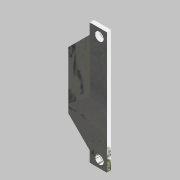
# Autodesk Inventor part: Tritt oben
Saved by Autodesk Inventor 2015 (Build 190159000, 159)
## iProperties
Created: 2017-04-11
Part Number: Tritt oben
Material: Generic
Document SubType Name: Modeling
Designer: Seelenernter
Density: 1 g/cm^3
Appearance: Chrom - poliert
Author: Seelenernter
Autodesk Inventor part; units mm, degrees
ref_plane "YZ Plane" through (0, 0, 0) normal (1, 0, 0) x (0, 1, 0)
sketch "Skizze1" plane through (0, 0, 0) normal (0, 1, 0) x (-1, 0, 0)
  line L0 (-90, 285) -> (90, 285)
  line L1 (90, 285) -> (90, -285)
  line L2 (90, -285) -> (-90, -285)
  line L3 (-90, -285) -> (-90, 285)
  line L4 (-90, 285) -> (90, -285) construction
  line L5 (90, 285) -> (-90, -285) construction
  point P0 (0, 0)
  dimension "d0" = 180
  dimension "d1" = 570
  constraints: 12 end point, 2 midpoint, 2 parallel, 1 horizontal, 1 perpendicular
  measures "d0" distance of L1.end L2.end
  measures "d1" distance of L0.end L1.end
extrude "Extrusion1" add sketch "Skizze1" along normal blind 20
sketch "Skizze2" plane through (0, 20, 0) normal (0, 1, 0) x (1, 0, 0)
  line L0 (-90, -285) -> (90, -285) projected
  line L1 (90, -285) -> (90, 285) projected
  line L2 (90, 285) -> (-90, 285) projected
  line L3 (-90, 285) -> (-90, -285) projected
  circle A0 centre (55, -250) radius 20
  point P0 (0, 0)
  dimension "d4" = 35
  dimension "d5" = 35
  dimension "d6" = 40
  constraints: 1 centre point
  measures "d4" distance from line of L1 A0.centre
  measures "d5" distance from line of L0 A0.centre
  measures "d6" diameter of A0
extrude "Extrusion2" cut sketch "Skizze2" against normal blind 20 contours A0
mirror "Spiegeln1" about plane through (0, 0, 0) normal (0, 0, 1) of "Extrusion2"
sketch "Skizze3" plane through (0, 20, 0) normal (0, 1, 0) x (1, 0, 0)
  circle A0 centre (25, -195) radius 5
  line L0 (-90, -285) -> (90, -285) projected
  line L1 (-90, 285) -> (-90, -285) projected
  circle A1 centre (75, -195) radius 5
  line L2 (90, -285) -> (90, 285) projected
  circle A2 centre (50, -165) radius 5
  circle A3 centre (50, -110) radius 5
  circle A4 centre (50, -55) radius 5
  circle A5 centre (50, 0) radius 5
  circle A6 centre (50, 55) radius 5
  circle A7 centre (50, 110) radius 5
  circle A8 centre (50, 165) radius 5
  circle A9 centre (25, -140) radius 5
  circle A10 centre (75, -140) radius 5
  circle A11 centre (25, -85) radius 5
  circle A12 centre (75, -85) radius 5
  circle A13 centre (25, -30) radius 5
  circle A14 centre (75, -30) radius 5
  circle A15 centre (25, 25) radius 5
  circle A16 centre (75, 25) radius 5
  circle A17 centre (25, 80) radius 5
  circle A18 centre (75, 80) radius 5
  circle A19 centre (25, 135) radius 5
  circle A20 centre (75, 135) radius 5
  circle A21 centre (25, 190) radius 5
  circle A22 centre (75, 190) radius 5
  point P0 (0, 0)
  dimension "d9" = 10
  dimension "d10" = 90
  dimension "d11" = 115
  dimension "d12" = 10
  dimension "d13" = 90
  dimension "d14" = 15
  dimension "d15" = 10
  dimension "d16" = 120
  dimension "d19" = 55
  dimension "d26" = 55
  dimension "d42" = 25
  constraints: 23 centre point, 2 vertical, 40 other
  measures "d9" diameter of A0
  measures "d10" distance from line of L0 A0.centre
  measures "d11" distance from line of A0.centre L1
  measures "d12" diameter of A1
  measures "d13" distance from line of L0 A1.centre
  measures "d14" distance from line of L2 A1.centre
  measures "d15" diameter of A2
  measures "d16" distance from line of L0 A2.centre
  measures "d19" distance of A2.centre A3.centre
  measures "d26" distance of A0.centre A9.centre
  measures "d42" horizontal distance of A1.centre A2.centre
extrude "Extrusion3" add sketch "Skizze3" along normal blind 2
fillet "Rundung1" radius 2 46 edges at (20, 22, 195) (20, 22, 140) (45, 22, 165) (70, 22, 195) (70, 22, 140) (45, 22, 110) (20, 22, 85) (70, 22, 85) (45, 22, 55) (20, 22, 30) (70, 22, 30) (45, 22, 0) (20, 22, -25) (70, 22, -25) (45, 22, -55) (20, 22, -80) (70, 22, -80) (45, 22, -110) (20, 22, -135) (70, 22, -135) (45, 22, -165) (20, 22, -190) (70, 22, -190) (70, 20, -190) (45, 20, -165) (20, 20, -190) (20, 20, -135) (45, 20, -110) (70, 20, -135) (20, 20, -80) (45, 20, -55) (70, 20, -80) (70, 20, -25) (45, 20, 0) (20, 20, -25) (20, 20, 30) (70, 20, 30) (45, 20, 55) (20, 20, 85) (45, 20, 110) (70, 20, 85) (70, 20, 140) (45, 20, 165) (20, 20, 140) (20, 20, 195) (70, 20, 195)
sketch "Skizze4" plane through (0, 20, 0) normal (0, 1, 0) x (1, 0, 0)
  line L0 (90, -285) -> (-90, -285) projected
  line L1 (13, -285) -> (13, 285)
  line L2 (-90, 285) -> (90, 285) projected
  line L3 (15, 285) -> (15, -285)
  point P0 (0, 0)
  dimension "d34" = 103
  dimension "d35" = 2
  constraints: 4 end point, 4 point on line, 1 parallel, 1 vertical
  measures "d34" distance from line of L0.end L1
  measures "d35" distance between parallel lines of L1 L3
extrude "Extrusion4" cut sketch "Skizze4" against normal blind 1
sketch "Skizze5" plane through (-90, 0, 285) normal (0, 0, 1) x (1, 0, 0)
  line L0 (103, 19) -> (103, 20) projected
  line L1 (0, 20) -> (103, 20) projected
  line L2 (0, 0) -> (0, 20) projected
  line L3 (180, 0) -> (0, 0) projected
  line L4 (180, 0) -> (180, 20) projected
  line L5 (105, 20) -> (180, 20) projected
  line L6 (105, 20) -> (105, 19) projected
  line L7 (105, 19) -> (103, 19) projected
  line L8 (103, 19) -> (103, 0)
  line L9 (0, 0) -> (180, 0) projected
  line L10 (105, 19) -> (105, 0)
  point P0 (90, 0)
  constraints: 4 end point, 2 point on line, 1 parallel, 1 vertical
extrude "Extrusion5" cut sketch "Skizze5" against normal blind 1 contours L7 L10 L3 L8
sketch "Skizze6" plane through (90, 0, -285) normal (0, 0, -1) x (-1, 0, 0)
  line L0 (77, 20) -> (77, 19) projected
  line L1 (77, 19) -> (75, 19) projected
  line L2 (75, 19) -> (75, 20) projected
  line L3 (0, 20) -> (75, 20) projected
  line L4 (0, 0) -> (0, 20) projected
  line L5 (180, 0) -> (0, 0) projected
  line L6 (180, 0) -> (180, 20) projected
  line L7 (77, 20) -> (180, 20) projected
  line L8 (75, 19) -> (75, 0)
  line L9 (77, 19) -> (77, 0)
  line L10 (180, 0) -> (0, 0) projected
  point P0 (90, 0)
  constraints: 4 end point, 1 perpendicular, 1 point on line, 1 vertical
extrude "Extrusion6" cut sketch "Skizze6" against normal blind 1 contours L9 L5 L8 L1
sketch "Skizze7" plane through (0, 20, 0) normal (0, 1, 0) x (1, 0, 0)
  line L0 (13, -285) -> (13, 285) projected
  line L1 (13, 285) -> (-90, 285) projected
  line L2 (-90, 285) -> (-90, -285) projected
  line L3 (-90, -285) -> (13, -285) projected
  line L4 (13, -285) -> (-90, -285) projected
  line L5 (10, -285) -> (10, -235)
  line L6 (10, -235) -> (-90, -135)
  line L7 (-90, 285) -> (-90, -285) projected
  line L8 (90, -285) -> (90, 285) projected
  point P0 (0, 0)
  dimension "d43" = 80
  dimension "d44" = 50
  dimension "d45" = 45
  constraints: 4 end point, 2 point on line, 1 parallel
  measures "d43" distance between parallel lines of L8 L5
  measures "d44" distance of L5.start L5.end
  measures "d45" angle of L5 L6
extrude "Extrusion7" cut sketch "Skizze7" against normal blind 20 contours L3 L2 L6 L5
ref_plane "Arbeitsebene1" through (0, 0, 0) normal (0, 0, 1) x (1, 0, 0)
mirror "Spiegeln2" about plane through (0, 0, 0) normal (0, 0, 1) of "Extrusion7"
ref_plane "Arbeitsebene2" through (0, 0, 285) normal (1, 0, 0) x (0, 0, -1)
sketch "Skizze9" plane through (0, 20, 0) normal (0, 1, 0) x (1, 0, 0)
  circle A0 centre (-75, -85) radius 5
  circle A1 centre (-50, -55) radius 5
  circle A2 centre (-25, -85) radius 5
  line L0 (-90, -135) -> (-90, 135) projected
  circle A3 centre (25, -85) radius 3 projected
  circle A4 centre (25, -85) radius 6.4641 projected
  circle A5 centre (50, -55) radius 6.4641 projected
  point P0 (0, 0)
  dimension "d50" = 10
  dimension "d51" = 10
  dimension "d52" = 10
  dimension "d53" = 15
  dimension "d55" = 25
  dimension "d56" = 25
  constraints: 3 centre point, 3 horizontal alignment
  measures "d50" diameter of A0
  measures "d51" diameter of A1
  measures "d52" diameter of A2
  measures "d53" distance from line of L0 A0.centre
  measures "d55" horizontal distance of A0.centre A1.centre
  measures "d56" horizontal distance of A1.centre A2.centre
extrude "Extrusion8" add sketch "Skizze9" along normal blind 2 contours A0 | A1 | A2
fillet "Rundung2" radius 2 6 edges at (-80, 22, 85) (-80, 20, 85) (-55, 22, 55) (-55, 20, 55) (-30, 22, 85) (-30, 20, 85)
pattern_linear "Rechteckige Anordnung1" count 2 spacing 55 along (0, 0, -1) of "Extrusion8", "Rundung2"
mirror "Spiegeln3" about plane through (0, 0, 0) normal (0, 0, 1) of "Extrusion8", "Rundung2"
sketch "Skizze10" plane through (0, 20, 0) normal (0, 1, 0) x (1, 0, 0)
  circle A0 centre (-75, 25) radius 5
  circle A1 centre (-25, 25) radius 5
  circle A2 centre (-50, 55) radius 6.4641 projected
  circle A3 centre (25, 25) radius 6.4641 projected
  circle A4 centre (-25, 85) radius 6.4641 projected
  circle A5 centre (-75, 85) radius 6.4641 projected
  point P0 (0, 0)
  dimension "d63" = 10
  dimension "d64" = 10
  constraints: 2 centre point, 2 horizontal alignment, 2 vertical alignment
  measures "d63" diameter of A0
  measures "d64" diameter of A1
extrude "Extrusion9" add sketch "Skizze10" along normal blind 2 contours A0 | A1
fillet "Rundung3" radius 2 4 edges at (-80, 22, -25) (-80, 20, -25) (-30, 22, -25) (-30, 20, -25)
sketch "Skizze11" plane through (0, 20, 0) normal (0, 1, 0) x (1, 0, 0)
  line L0 (10, -235) -> (-90, -135) projected
  line L1 (-10.9204, -214.0796) -> (-10.9204, 214.0796)
  line L2 (-90, 135) -> (10, 235) projected
  line L3 (-9.9204, -215.0796) -> (-9.9204, 215.0796)
  point P0 (0, 0)
  dimension "d68" = 1
  constraints: 4 end point, 4 point on line, 1 parallel, 1 vertical
  measures "d68" distance between parallel lines of L1 L3
extrude "Extrusion10" cut sketch "Skizze11" against normal blind 1
